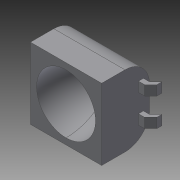
# Autodesk Inventor part: top
Saved by Autodesk Inventor 2014 SP2 (Build 180246200, 246)
## iProperties
Created: 2014-11-27
Part Number: top
Material: Generic
Document SubType Name: Modeling
Designer: No
Density: 1 g/cm^3
Appearance: Default
Author: No
Autodesk Inventor part; units mm, degrees
ref_plane "XZ Plane" through (0, 0, 0) normal (0, 1, 0) x (-1, 0, 0)
sketch "Sketch1" plane through (0, 0, 0) normal (0, 1, 0) x (-1, 0, 0)
  line L0 (-29, 29) -> (29, 29)
  line L1 (29, 29) -> (29, -29)
  line L2 (29, -29) -> (-29, -29)
  line L3 (-29, -29) -> (-29, 29)
  line L4 (-29, 29) -> (29, -29) construction
  line L5 (29, 29) -> (-29, -29) construction
  point P0 (0, 0)
  dimension "d0" = 58
  dimension "d1" = 58
  constraints: 12 end point, 2 midpoint, 2 parallel, 1 horizontal, 1 perpendicular
  measures "d0" distance of L1.end L2.end
  measures "d1" distance of L0.end L1.end
extrude "Extrusion1" add sketch "Sketch1" along normal blind 39
sketch "Sketch2" plane through (0, 0, 0) normal (1, 0, 0) x (0, 1, 0)
  line L0 (0, 0) -> (33, 0) construction
  ellipse E0 centre (0, 0) end of major axis (33, 0) minor radius 24 (-33, 0) -> (33, 0) ccw
  line L1 (-33, 0) -> (33, 0)
  line L2 (53.4, 0) -> (-47.4, 0) projected
  dimension "d6" = 24
  dimension "d5" = 33
  constraints: 4 end point, 3 horizontal, 1 coincident, 4 other
  measures "d5" distance of L0.start L0.end
revolve "Revolution1" cut sketch "Sketch2" angle 360 about axis through (0, 0, 0) along (0, -1, 0)
sketch "Sketch3" plane through (29, 0, 29) normal (1, 0, 0) x (0, 0, -1)
  line L0 (0, 0) -> (0, 39) projected
  line L1 (29, 59.7326) -> (29, -35.1874)
  line L2 (13.5, 34) -> (21.5, 34)
  line L3 (21.5, 34) -> (21.5, 30)
  line L4 (21.5, 30) -> (13.5, 30)
  line L5 (13.5, 30) -> (13.5, 34)
  line L6 (13.5, 34) -> (21.5, 30) construction
  line L7 (21.5, 34) -> (13.5, 30) construction
  line L8 (0, 39) -> (58, 39) projected
  point P0 (29, 0)
  point P1 (17.5, 32)
  dimension "d8" = 8
  dimension "d9" = 4
  dimension "d10" = 15
  dimension "d14" = 5
  constraints: 14 end point, 3 parallel, 2 midpoint, 1 horizontal, 1 perpendicular, 1 vertical
  measures "d8" distance of L3.end L4.end
  measures "d9" distance of L2.end L3.end
  measures "d10" diameter of L3 L1
  measures "d14" distance between parallel lines of L8 L2
extrude "Extrusion2" add sketch "Sketch3" along normal blind 5
sketch "Sketch6" plane through (29, 30, 15.5) normal (0, 0, 1) x (1, 0, 0)
  line L0 (5, 4) -> (5, 0) projected
  line L1 (0, -30) -> (-58, -30) projected
  line L2 (0, -30) -> (0, 9) projected
  line L3 (-58, 9) -> (0, 9) projected
  line L4 (-58, -30) -> (-58, 9) projected
  line L5 (5, 4) -> (10, 9)
  line L6 (5, 4) -> (12.0711, 4) construction
  line L7 (10, 9) -> (10, 5)
  line L8 (10, 5) -> (5, 0)
  point P0 (-29, -30)
  dimension "d18" = 45
  dimension "d19" = 4
  constraints: 8 end point, 1 equal length, 1 horizontal, 1 perpendicular
  measures "d18" angle of L6 L5
  measures "d19" distance of L5.end L7.end
extrude "Extrusion3" add sketch "Sketch6" against normal up to surface (8 mm away) contours L5 L7 L8 L0
mirror "Mirror1" about plane through (0, 0, 0) normal (0, 0, 1) of "Extrusion2", "Extrusion3"
mirror "Mirror2" about plane through (0, 0, 0) normal (1, 0, 0) of "Extrusion3", "Extrusion2", "Mirror1"
fillet "Fillet1" radius 20 2 edges at (0, 39, 29) (0, 39, -29)
equation "\"d19\" = d9"
body "Solid1"
